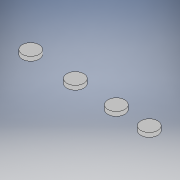
# Autodesk Inventor part: VacuumWheels
Saved by Autodesk Inventor 2018 (Build 220112000, 112)
## iProperties
Created: 2019-01-08
Part Number: VacuumWheels
Material: Generic
Document SubType Name: Modeling
Designer: Gabriel
Density: 1 g/cm^3
Appearance: Default
Author: Gabriel
Autodesk Inventor part; units mm, degrees
ref_plane "YZ Plane" through (0, 0, 0) normal (1, 0, 0) x (0, 1, 0)
ref_plane "XZ Plane" through (0, 0, 0) normal (0, 1, 0) x (-1, 0, 0)
ref_plane "XY Plane" through (0, 0, 0) normal (0, 0, 1) x (1, 0, 0)
sketch "Sketch1" plane through (0, 0, 0) normal (0, 1, 0) x (-1, 0, 0)
  circle A0 centre (86.2847, -78.375) radius 50.8
  circle A1 centre (86.2847, -78.375) radius 12.7
  dimension "d0" = 101.6
  dimension "d12" = 38.1
  constraints: 2 centre point
  measures "d0" diameter of A0
  measures "d12" radial gap between concentric circles of A0 A1
extrude "Extrusion4" add sketch "Sketch1" along normal blind 25.4
body "Solid4"
